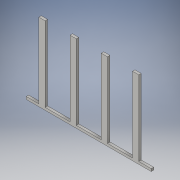
# Autodesk Inventor part: Bucket - Rake
Saved by Autodesk Inventor 2016 (Build 200138000, 138)
## iProperties
Created: 2015-12-17
Part Number: Bucket - Rake
Material: Generic
Document SubType Name: Modeling
Designer: TimB
Density: 1 g/cm^3
Appearance: Default
Author: TimB
Autodesk Inventor part; units mm, degrees
ref_plane "YZ Plane" through (0, 0, 0) normal (1, 0, 0) x (0, 1, 0)
ref_plane "XZ Plane" through (0, 0, 0) normal (0, 1, 0) x (-1, 0, 0)
ref_plane "XY Plane" through (0, 0, 0) normal (0, 0, 1) x (1, 0, 0)
sketch "Sketch1" plane through (0, 0, 0) normal (0, 0, 1) x (1, 0, 0)
  line L0 (-149.3708, -1.27) -> (-22.3708, -1.27)
  line L1 (-22.3708, -1.27) -> (-22.3708, 1.27)
  line L2 (-149.3708, 1.27) -> (-149.3708, -1.27)
  line L3 (-149.3708, -1.27) -> (-22.3708, 1.27) construction
  line L4 (-22.3708, -1.27) -> (-149.3708, 1.27) construction
  line L5 (-149.3708, 1.27) -> (-136.6708, 1.27)
  line L6 (-22.3708, 1.27) -> (-35.0708, 1.27)
  line L7 (-130.3208, 1.27) -> (-130.3208, 77.47)
  line L8 (-130.3208, 77.47) -> (-136.6708, 77.47)
  line L9 (-136.6708, 77.47) -> (-136.6708, 1.27)
  line L10 (-130.3208, 1.27) -> (-104.9208, 1.27)
  line L11 (-98.5708, 1.27) -> (-98.5708, 77.47)
  line L12 (-98.5708, 77.47) -> (-104.9208, 77.47)
  line L13 (-104.9208, 77.47) -> (-104.9208, 1.27)
  line L14 (-41.4208, 1.27) -> (-41.4208, 77.47)
  line L15 (-41.4208, 77.47) -> (-35.0708, 77.47)
  line L16 (-35.0708, 77.47) -> (-35.0708, 1.27)
  line L17 (-41.4208, 1.27) -> (-66.8208, 1.27)
  line L18 (-73.1708, 1.27) -> (-73.1708, 77.47)
  line L19 (-73.1708, 77.47) -> (-66.8208, 77.47)
  line L20 (-66.8208, 77.47) -> (-66.8208, 1.27)
  line L21 (-98.5708, 1.27) -> (-73.1708, 1.27)
  point P0 (0, 0)
  point P1 (-85.8708, 0)
  dimension "d0" = 127
  dimension "d1" = 2.54
  dimension "d2" = 12.7
  dimension "d3" = 12.7
  dimension "d4" = 6.35
  dimension "d5" = 76.2
  dimension "d6" = 25.4
  dimension "d7" = 6.35
  dimension "d8" = 6.35
  dimension "d9" = 76.2
  dimension "d10" = 25.4
  dimension "d11" = 6.35
  dimension "d12" = 76.2
  constraints: 44 end point, 5 parallel, 2 midpoint, 2 perpendicular, 1 horizontal
  measures "d0" distance of L2.start L1.end
  measures "d1" distance of L1.end L0.end
  measures "d2" distance of L2.start L5.end
  measures "d3" distance of L1.end L6.end
  measures "d4" distance of L8.end L7.end
  measures "d5" distance of L7.end L7.start
  measures "d6" distance of L7.start L10.end
  measures "d7" distance of L12.end L11.end
  measures "d8" distance of L14.end L15.end
  measures "d9" distance of L14.start L14.end
  measures "d10" distance of L14.start L17.end
  measures "d11" distance of L18.end L19.end
  measures "d12" distance of L18.start L18.end
extrude "Extrusion1" add sketch "Sketch1" along normal blind 2.54
body "Solid1"
